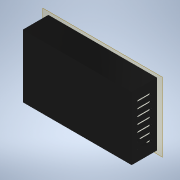
# Autodesk Inventor part: HANDHELD_BOTTOM
Saved by Autodesk Inventor 2020 (Build 240168000, 168)
## iProperties
Created: 2023-03-16
Part Number: HANDHELD_BOTTOM
Material: PC/ABS Plastic
Document SubType Name: Modeling
Designer: catsm
Density: 0.357273 g/cm^3
Appearance: Smooth - White
Author: catsm
Autodesk Inventor part; units mm, degrees
ref_plane "YZ Plane" through (0, 0, 0) normal (1, 0, 0) x (0, 1, 0)
ref_plane "XZ Plane" through (0, 0, 0) normal (0, 1, 0) x (-1, 0, 0)
ref_plane "Work Plane1" through (0, 0, 0) normal (0, 0, 1) x (1, 0, 0)
sketch "Sketch1" plane through (0, 0, 0) normal (0, 0, 1) x (1, 0, 0)
  line L0 (-101.8665, 59.0165) -> (-101.8665, -59.0165) projected
  line L1 (101.8665, 59.0165) -> (-101.8665, 59.0165) projected
  line L2 (101.8665, -59.0165) -> (101.8665, 59.0165) projected
  line L3 (-101.8665, -59.0165) -> (101.8665, -59.0165) projected
  line L4 (-98.6915, 55.8415) -> (-98.6915, -55.8415)
  line L5 (-98.6915, -55.8415) -> (98.6915, -55.8415)
  line L6 (98.6915, -55.8415) -> (98.6915, 55.8415)
  line L7 (98.6915, 55.8415) -> (-98.6915, 55.8415)
  point P0 (0, 0)
  dimension "d0" = 3.175
  constraints: 8 end point, 3 other
  measures "d0" distance between parallel lines of L1 L7
extrude "Extrusion1" add sketch "Sketch1" along normal blind 44.45
sketch "Sketch2" plane through (101.8665, -59.0165, 0) normal (1, 0, 0) x (0, 0, -1)
  circle A0 centre (-3.048, 109.9558) radius 1.905 projected
  circle A1 centre (-3.048, 8.0772) radius 1.778 projected
  circle A2 centre (-3.048, 8.0772) radius 1.016
  circle A3 centre (-3.048, 109.9558) radius 1.016
  point P0 (0, 59.0165)
  dimension "d3" = 2.032
  dimension "d4" = 2.032
  constraints: 2 centre point, 2 coincident
  measures "d3" diameter of A2
  measures "d4" diameter of A3
extrude "Extrusion2" cut sketch "Sketch2" against normal up to surface (203.733 mm away) contours A2 | A3
sketch "Sketch3" plane through (0, 0, 44.45) normal (0, 0, 1) x (1, 0, 0)
  line L0 (101.8665, 59.0165) -> (-101.8665, 59.0165) projected
  line L1 (-101.8665, 59.0165) -> (-101.8665, -59.0165) projected
  line L2 (-101.8665, -59.0165) -> (101.8665, -59.0165) projected
  line L3 (101.8665, -59.0165) -> (101.8665, 59.0165) projected
  line L4 (-98.6915, 55.8415) -> (98.6915, 55.8415) projected
  line L5 (98.6915, 55.8415) -> (98.6915, -55.8415) projected
  line L6 (98.6915, -55.8415) -> (-98.6915, -55.8415) projected
  line L7 (-98.6915, -55.8415) -> (-98.6915, 55.8415) projected
  point P0 (0, 0)
extrude "Extrusion3" add sketch "Sketch3" along normal blind 3.175 contours L3 L2 L1 L0 | L4 L5 L6 L7
sketch "Sketch4" plane through (0, 0, 44.45) normal (0, 0, -1) x (-1, 0, 0)
  circle A0 centre (93.7487, 50.8987) radius 1.5 projected
  circle A1 centre (93.7487, -40.5657) radius 1.5 projected
  circle A2 centre (38.7843, -40.5657) radius 1.5 projected
  circle A3 centre (38.7843, 50.8987) radius 1.5 projected
  circle A4 centre (93.7487, 50.8987) radius 3.556
  circle A5 centre (38.7843, 50.8987) radius 3.556
  circle A6 centre (38.7843, -40.5657) radius 3.556
  circle A7 centre (93.7487, -40.5657) radius 3.556
  point P0 (0, 0)
  dimension "d9" = 7.112
  dimension "d22" = 7.112
  dimension "d23" = 7.112
  dimension "d24" = 7.112
  constraints: 4 centre point, 1 coincident
  measures "d9" diameter of A4
  measures "d22" diameter of A5
  measures "d23" diameter of A6
  measures "d24" diameter of A7
ref_plane "Work Plane2" through (37.0165, -42.3335, 36.6431) normal (0, 0, 1) x (1, 0, 0)
extrude "Extrusion4" add sketch "Sketch4" along normal up to surface (7.8069 mm away) contours A0 | A1 | A2 | A3 | A4 | A5 | A6 | A7
sketch "Sketch6" plane through (-38.7843, -40.5657, 36.6431) normal (0, 0, -1) x (-1, 0, 0)
  circle A0 centre (0, 0) radius 1.5 projected
  circle A1 centre (54.9645, 0) radius 1.5 projected
  circle A2 centre (54.9645, 91.4645) radius 1.5 projected
  circle A3 centre (0, 91.4645) radius 1.5 projected
  circle A4 centre (54.9645, 91.4645) radius 3.556 projected
  point P0 (-38.7843, 40.5657)
  constraints: 4 coincident
hole "Hole2" at (-93.7487, 50.8987, 36.6431) at (-38.7843, 50.8987, 36.6431) at (-38.7843, -40.5657, 36.6431) at (-93.7487, -40.5657, 36.6431) direction (0, 0, 1) diameter 3.556 depth 7.8069 countersink diameter 3.81 countersink angle 82
sketch "Sketch7" plane through (0, 0, 44.45) normal (0, 0, -1) x (-1, 0, 0)
  line L0 (22.0258, -44.3326) -> (21.8153, -44.3326) projected
  line L1 (22.3278, -44.8451) -> (22.3278, -44.6284) projected
  line L2 (15.6236, -51.3326) -> (15.8403, -51.3326) projected
  line L3 (15.3278, -50.8201) -> (15.3278, -51.0306) projected
  line L4 (22.3278, -44.3326) -> (15.3278, -44.3326)
  line L5 (15.3278, -44.3326) -> (15.3278, -51.3326)
  line L6 (15.3278, -51.3326) -> (22.3278, -51.3326)
  line L7 (22.3278, -51.3326) -> (22.3278, -44.3326)
  line L8 (23.3044, -47.8326) -> (14.4144, -47.8326) construction
  line L9 (23.3044, -44.6576) -> (14.4144, -44.6576)
  line L10 (14.4144, -51.0076) -> (23.3044, -51.0076)
  arc A0 (23.3044, -51.0076) -> (23.3044, -44.6576) centre (23.3044, -47.8326) ccw
  arc A1 (14.4144, -44.6576) -> (14.4144, -51.0076) centre (14.4144, -47.8326) ccw
  line L11 (26.4794, -38.1722) -> (26.4794, -56.2222) projected
  line L12 (11.2394, -56.2222) -> (11.2394, -38.1722) projected
  point P0 (0, 0)
  point P1 (18.8594, -47.8326)
  dimension "d32" = 6.35
  dimension "d33" = 3.175
  dimension "d34" = 3.175
  constraints: 16 end point, 4 point on circle, 4 tangent, 3 parallel, 2 centre point, 2 perpendicular, 1 horizontal, 1 midpoint
  measures "d32" diameter of A1
  measures "d33" distance from line of L11 L8.start
  measures "d34" distance from line of L12 L8.end
extrude "Extrusion5" add sketch "Sketch7" along normal blind 6.35 contours L9 L1 L7 L10 L3 L5 | L5 L3 L10 A1 L9 | L9 A0 L10 L7 L1
sketch "Sketch8" plane through (-98.6915, -55.8415, 0) normal (0, 1, 0) x (1, 0, 0)
  line L0 (87.4521, -37.1) -> (87.4521, -35.5) projected
  line L1 (86.9521, -35.5) -> (72.7121, -35.5) projected
  line L2 (86.9521, -37.1) -> (72.7121, -37.1) projected
  line L3 (72.2121, -37.1) -> (72.2121, -35.5) projected
  line L4 (87.4521, -35.5) -> (87.4521, -37.1) projected
  line L5 (72.2121, -35.5) -> (87.4521, -35.5)
  line L6 (87.4521, -35.5) -> (87.4521, -37.1)
  line L7 (87.4521, -37.1) -> (72.2121, -37.1)
  line L8 (72.2121, -37.1) -> (72.2121, -35.5)
  line L9 (87.7061, -35.246) -> (71.9581, -35.246)
  line L10 (71.9581, -35.246) -> (71.9581, -37.354)
  line L11 (71.9581, -37.354) -> (87.7061, -37.354)
  line L12 (87.7061, -37.354) -> (87.7061, -35.246)
  point P0 (98.6915, 0)
  dimension "d37" = 0.254
  constraints: 16 end point, 4 parallel, 2 perpendicular, 1 horizontal, 3 other
  measures "d37" distance between parallel lines of L5 L9
extrude "Extrusion6" cut sketch "Sketch8" against normal blind 1.143 contours L7 L2 L3 L5 L1 L0 | L12 L11 L10 L9
sketch "Sketch9" plane through (-101.8665, -59.0165, 0) normal (0, -1, 0) x (1, 0, 0)
  line L0 (89.9919, 33.75) -> (89.9919, 35.4) projected
  line L1 (75.9919, 33.75) -> (75.9919, 35.4) projected
  line L2 (77.3919, 33.65) -> (76.0919, 33.65) projected
  line L3 (76.1819, 35.5) -> (77.3919, 35.5) projected
  line L4 (75.9919, 35.5) -> (89.9919, 35.5)
  line L5 (89.9919, 35.5) -> (89.9919, 33.65)
  line L6 (89.9919, 33.65) -> (75.9919, 33.65)
  line L7 (75.9919, 33.65) -> (75.9919, 35.5)
  line L8 (75.7379, 33.396) -> (90.2459, 33.396)
  line L9 (90.2459, 33.396) -> (90.2459, 35.754)
  line L10 (90.2459, 35.754) -> (75.7379, 35.754)
  line L11 (75.7379, 35.754) -> (75.7379, 33.396)
  point P0 (101.8665, 0)
  dimension "d40" = 0.254
  constraints: 16 end point, 4 parallel, 2 perpendicular, 2 point on line, 1 horizontal, 3 other
  measures "d40" distance between parallel lines of L6 L8
extrude "Extrusion7" cut sketch "Sketch9" against normal up to surface (3.175 mm away) contours L5 L6 L2 L7 L1 L4 L3 L0 | L11 L10 L9 L8
sketch "Sketch10" plane through (-101.8665, -59.0165, 0) normal (0, -1, 0) x (1, 0, 0)
  line L0 (90.2459, 35.754) -> (90.2459, 33.396) projected
  line L1 (90.2459, 33.396) -> (75.7379, 33.396) projected
  line L2 (75.7379, 33.396) -> (75.7379, 35.754) projected
  line L3 (75.7379, 35.754) -> (90.2459, 35.754) projected
  line L4 (0, 0) -> (203.733, 0) projected
  line L5 (203.733, 0) -> (203.733, 47.625) projected
  line L6 (0, 47.625) -> (203.733, 47.625) projected
  line L7 (0, 0) -> (0, 47.625) projected
  line L8 (72.5629, 30.221) -> (93.4209, 30.221)
  line L9 (93.4209, 30.221) -> (93.4209, 38.929)
  line L10 (93.4209, 38.929) -> (72.5629, 38.929)
  line L11 (72.5629, 38.929) -> (72.5629, 30.221)
  point P0 (101.8665, 0)
  dimension "d43" = 3.175
  constraints: 8 end point, 3 other
  measures "d43" distance between parallel lines of L1 L8
extrude "Extrusion8" cut sketch "Sketch10" against normal blind 1.5875 contours L11 L10 L9 L8
sketch "Sketch11" plane through (0, 0, 44.45) normal (0, 0, -1) x (-1, 0, 0)
  line L0 (-82.4355, -55.2065) -> (-82.4355, -39.2045) projected
  line L1 (-92.3415, -39.2045) -> (-92.3415, -55.2065) projected
  line L2 (-84.023, -48.412) -> (-90.754, -48.412) construction
  line L3 (-84.023, -46.8245) -> (-90.754, -46.8245)
  line L4 (-90.754, -49.9995) -> (-84.023, -49.9995)
  arc A0 (-84.023, -49.9995) -> (-84.023, -46.8245) centre (-84.023, -48.412) ccw
  arc A1 (-90.754, -46.8245) -> (-90.754, -49.9995) centre (-90.754, -48.412) ccw
  line L5 (-98.6915, 55.8415) -> (-98.6915, -55.8415) projected
  line L6 (-98.6915, -55.8415) -> (98.6915, -55.8415) projected
  point P0 (0, 0)
  point P1 (-87.3885, -48.412)
  dimension "d49" = 1.5875
  dimension "d50" = 1.5875
  dimension "d51" = 1.5875
  dimension "d52" = 7.62
  dimension "d92" = 7.9375
  dimension "d93" = 7.4295
  constraints: 8 end point, 4 point on circle, 4 tangent, 2 centre point, 1 horizontal, 1 midpoint, 1 parallel
  measures "d49" distance from line of L1 L2.end
  measures "d50" distance from line of L0 L2.start
  measures "d51" radius of A0
  measures "d52" distance from line of L1.start L3
  measures "d92" distance from line of L5 L2.end
  measures "d93" distance from line of L6 L2.end
extrude "Extrusion9" add sketch "Sketch11" along normal blind 6.35
sketch "Sketch17" plane through (-101.8665, -59.0165, 0) normal (0, -1, 0) x (1, 0, 0)
  line L0 (184.8894, 33.1978) -> (193.6206, 33.1978) projected
  line L1 (193.6206, 36.3728) -> (184.8894, 36.3728) projected
  line L2 (193.6206, 33.1978) -> (193.6206, 36.3728) projected
  line L3 (72.5629, 30.221) -> (72.5629, 38.929) projected
  line L4 (72.5629, 38.929) -> (93.4209, 38.929) projected
  line L5 (93.4209, 38.929) -> (93.4209, 30.221) projected
  line L6 (93.4209, 30.221) -> (72.5629, 30.221) projected
  line L7 (0, 0) -> (203.733, 0) projected
  line L8 (203.733, 0) -> (203.733, 47.625) projected
  line L9 (0, 47.625) -> (203.733, 47.625) projected
  line L10 (0, 0) -> (0, 47.625) projected
  line L11 (184.8894, 36.3728) -> (184.8894, 33.1978) projected
  line L12 (184.302, 38.1) -> (184.302, 36.5252) projected
  line L13 (194.208, 38.1) -> (194.208, 36.5252) projected
  line L14 (194.208, 38.1) -> (184.302, 38.1) projected
  line L15 (193.8746, 32.9438) -> (184.6354, 32.9438)
  line L16 (184.6354, 32.9438) -> (184.6354, 36.6268)
  line L17 (184.6354, 36.6268) -> (193.8746, 36.6268)
  line L18 (193.8746, 36.6268) -> (193.8746, 32.9438)
  point P0 (101.8665, 0)
  dimension "d74" = 0.254
  constraints: 8 end point, 3 other
  measures "d74" distance between parallel lines of L0 L15
extrude "Extrusion15" cut sketch "Sketch17" against normal up to surface (3.175 mm away) contours L11 L1 L2 L0 | L15 L16 L17 L18
sketch "Sketch18" plane through (-101.8665, -59.0165, 0) normal (0, -1, 0) x (1, 0, 0)
  line L0 (184.6354, 36.6268) -> (193.8746, 36.6268) projected
  line L1 (193.8746, 36.6268) -> (193.8746, 32.9438) projected
  line L2 (193.8746, 32.9438) -> (184.6354, 32.9438) projected
  line L3 (184.6354, 32.9438) -> (184.6354, 36.6268) projected
  line L4 (72.5629, 30.221) -> (72.5629, 38.929) projected
  line L5 (72.5629, 38.929) -> (93.4209, 38.929) projected
  line L6 (93.4209, 38.929) -> (93.4209, 30.221) projected
  line L7 (93.4209, 30.221) -> (72.5629, 30.221) projected
  line L8 (0, 0) -> (203.733, 0) projected
  line L9 (203.733, 0) -> (203.733, 47.625) projected
  line L10 (0, 47.625) -> (203.733, 47.625) projected
  line L11 (0, 0) -> (0, 47.625) projected
  line L12 (183.0479, 31.3563) -> (195.4621, 31.3563)
  line L13 (195.4621, 31.3563) -> (195.4621, 38.2143)
  line L14 (195.4621, 38.2143) -> (183.0479, 38.2143)
  line L15 (183.0479, 38.2143) -> (183.0479, 31.3563)
  point P0 (101.8665, 0)
  dimension "d77" = 1.5875
  constraints: 8 end point, 3 other
  measures "d77" distance between parallel lines of L2 L12
extrude "Extrusion16" cut sketch "Sketch18" against normal blind 1.5875 contours L15 L14 L13 L12
sketch "Sketch19" plane through (-101.8665, -59.0165, 0) normal (0, -1, 0) x (1, 0, 0)
  line L0 (183.0479, 31.3563) -> (183.0479, 38.2143) projected
  line L1 (184.6354, 36.6268) -> (184.6354, 32.9438) projected
  line L2 (184.6354, 36.6268) -> (184.6354, 32.9438) projected
  line L3 (184.6354, 34.7853) -> (183.0479, 34.7853)
  line L4 (183.0479, 31.3563) -> (183.0479, 38.2143) projected
  circle A0 centre (176.6979, 34.7853) radius 2.54
  circle A1 centre (167.1729, 34.7853) radius 2.54
  circle A2 centre (157.6479, 34.7853) radius 3.175
  point P0 (101.8665, 0)
  dimension "d80" = 5.08
  dimension "d81" = 5.08
  dimension "d82" = 6.35
  dimension "d83" = 0
  dimension "d84" = 6.35
  dimension "d85" = 9.525
  dimension "d86" = 9.525
  constraints: 3 centre point, 2 end point, 2 horizontal alignment, 2 midpoint
  measures "d80" diameter of A0
  measures "d81" diameter of A1
  measures "d82" diameter of A2
  measures "d83" distance from line of L3 A0.centre
  measures "d84" distance from line of L0 A0.centre
  measures "d85" distance of A1.centre A0.centre
  measures "d86" distance of A1.centre A2.centre
extrude "Extrusion17" cut sketch "Sketch19" against normal up to surface (3.175 mm away)
sketch "Sketch20" plane through (-101.8665, -59.0165, 0) normal (0, -1, 0) x (1, 0, 0)
  circle A0 centre (157.6479, 34.7853) radius 3.175 projected
  circle A1 centre (157.6479, 34.7853) radius 5.715
  point P0 (101.8665, 0)
  dimension "d89" = 2.54
  constraints: 1 centre point
  measures "d89" radial gap between concentric circles of A0 A1
extrude "Extrusion18" cut sketch "Sketch20" against normal blind 1.5875
sketch "Sketch21" plane through (101.8665, -59.0165, 0) normal (1, 0, 0) x (0, 0, -1)
  line L0 (-34.925, 59.0165) -> (-12.7, 59.0165) construction
  line L1 (-34.925, 56.4765) -> (-12.7, 56.4765)
  line L2 (-12.7, 61.5565) -> (-34.925, 61.5565)
  arc A0 (-34.925, 61.5565) -> (-34.925, 56.4765) centre (-34.925, 59.0165) ccw
  arc A1 (-12.7, 56.4765) -> (-12.7, 61.5565) centre (-12.7, 59.0165) ccw
  line L3 (0, 0) -> (0, 118.033) projected
  line L4 (-47.625, 0) -> (-47.625, 118.033) projected
  circle A2 centre (-3.048, 109.9558) radius 1.016 projected
  circle A3 centre (-3.048, 8.0772) radius 1.016 projected
  line L5 (0, 0) -> (0, 118.033) projected
  line L6 (0, 118.033) -> (-47.625, 118.033) projected
  line L7 (-47.625, 0) -> (-47.625, 118.033) projected
  line L8 (0, 0) -> (-47.625, 0) projected
  line L9 (-34.925, 69.1765) -> (-12.7, 69.1765)
  arc A4 (-12.7, 69.1765) -> (-12.7, 74.2565) centre (-12.7, 71.7165) ccw
  line L10 (-12.7, 74.2565) -> (-34.925, 74.2565)
  arc A5 (-34.925, 74.2565) -> (-34.925, 69.1765) centre (-34.925, 71.7165) ccw
  line L11 (-34.925, 81.8765) -> (-12.7, 81.8765)
  arc A6 (-12.7, 81.8765) -> (-12.7, 86.9565) centre (-12.7, 84.4165) ccw
  line L12 (-12.7, 86.9565) -> (-34.925, 86.9565)
  arc A7 (-34.925, 86.9565) -> (-34.925, 81.8765) centre (-34.925, 84.4165) ccw
  line L13 (-34.925, 94.5765) -> (-12.7, 94.5765)
  arc A8 (-12.7, 94.5765) -> (-12.7, 99.6565) centre (-12.7, 97.1165) ccw
  line L14 (-12.7, 99.6565) -> (-34.925, 99.6565)
  arc A9 (-34.925, 99.6565) -> (-34.925, 94.5765) centre (-34.925, 97.1165) ccw
  line L15 (-34.925, 43.7765) -> (-12.7, 43.7765)
  arc A10 (-12.7, 43.7765) -> (-12.7, 48.8565) centre (-12.7, 46.3165) ccw
  line L16 (-12.7, 48.8565) -> (-34.925, 48.8565)
  arc A11 (-34.925, 48.8565) -> (-34.925, 43.7765) centre (-34.925, 46.3165) ccw
  line L17 (-34.925, 56.4765) -> (-12.7, 56.4765)
  arc A12 (-12.7, 56.4765) -> (-12.7, 61.5565) centre (-12.7, 59.0165) ccw
  line L18 (-12.7, 61.5565) -> (-34.925, 61.5565)
  arc A13 (-34.925, 61.5565) -> (-34.925, 56.4765) centre (-34.925, 59.0165) ccw
  line L19 (-34.925, 69.1765) -> (-12.7, 69.1765)
  arc A14 (-12.7, 69.1765) -> (-12.7, 74.2565) centre (-12.7, 71.7165) ccw
  line L20 (-12.7, 74.2565) -> (-34.925, 74.2565)
  arc A15 (-34.925, 74.2565) -> (-34.925, 69.1765) centre (-34.925, 71.7165) ccw
  line L21 (-34.925, 81.8765) -> (-12.7, 81.8765)
  arc A16 (-12.7, 81.8765) -> (-12.7, 86.9565) centre (-12.7, 84.4165) ccw
  line L22 (-12.7, 86.9565) -> (-34.925, 86.9565)
  arc A17 (-34.925, 86.9565) -> (-34.925, 81.8765) centre (-34.925, 84.4165) ccw
  line L23 (-34.925, 31.0765) -> (-12.7, 31.0765)
  arc A18 (-12.7, 31.0765) -> (-12.7, 36.1565) centre (-12.7, 33.6165) ccw
  line L24 (-12.7, 36.1565) -> (-34.925, 36.1565)
  arc A19 (-34.925, 36.1565) -> (-34.925, 31.0765) centre (-34.925, 33.6165) ccw
  line L25 (-34.925, 43.7765) -> (-12.7, 43.7765)
  arc A20 (-12.7, 43.7765) -> (-12.7, 48.8565) centre (-12.7, 46.3165) ccw
  line L26 (-12.7, 48.8565) -> (-34.925, 48.8565)
  arc A21 (-34.925, 48.8565) -> (-34.925, 43.7765) centre (-34.925, 46.3165) ccw
  line L27 (-34.925, 56.4765) -> (-12.7, 56.4765)
  arc A22 (-12.7, 56.4765) -> (-12.7, 61.5565) centre (-12.7, 59.0165) ccw
  line L28 (-12.7, 61.5565) -> (-34.925, 61.5565)
  arc A23 (-34.925, 61.5565) -> (-34.925, 56.4765) centre (-34.925, 59.0165) ccw
  line L29 (-34.925, 69.1765) -> (-12.7, 69.1765)
  arc A24 (-12.7, 69.1765) -> (-12.7, 74.2565) centre (-12.7, 71.7165) ccw
  line L30 (-12.7, 74.2565) -> (-34.925, 74.2565)
  arc A25 (-34.925, 74.2565) -> (-34.925, 69.1765) centre (-34.925, 71.7165) ccw
  line L31 (-34.925, 18.3765) -> (-12.7, 18.3765)
  arc A26 (-12.7, 18.3765) -> (-12.7, 23.4565) centre (-12.7, 20.9165) ccw
  line L32 (-12.7, 23.4565) -> (-34.925, 23.4565)
  arc A27 (-34.925, 23.4565) -> (-34.925, 18.3765) centre (-34.925, 20.9165) ccw
  line L33 (-34.925, 31.0765) -> (-12.7, 31.0765)
  arc A28 (-12.7, 31.0765) -> (-12.7, 36.1565) centre (-12.7, 33.6165) ccw
  line L34 (-12.7, 36.1565) -> (-34.925, 36.1565)
  arc A29 (-34.925, 36.1565) -> (-34.925, 31.0765) centre (-34.925, 33.6165) ccw
  line L35 (-34.925, 43.7765) -> (-12.7, 43.7765)
  arc A30 (-12.7, 43.7765) -> (-12.7, 48.8565) centre (-12.7, 46.3165) ccw
  line L36 (-12.7, 48.8565) -> (-34.925, 48.8565)
  arc A31 (-34.925, 48.8565) -> (-34.925, 43.7765) centre (-34.925, 46.3165) ccw
  line L37 (-34.925, 56.4765) -> (-12.7, 56.4765)
  arc A32 (-12.7, 56.4765) -> (-12.7, 61.5565) centre (-12.7, 59.0165) ccw
  line L38 (-12.7, 61.5565) -> (-34.925, 61.5565)
  arc A33 (-34.925, 61.5565) -> (-34.925, 56.4765) centre (-34.925, 59.0165) ccw
  point P0 (0, 59.0165)
  point P1 (-23.8125, 59.0165)
  dimension "d95" = 5.08
  dimension "d96" = 12.7
  dimension "d97" = 12.7
  dimension "d98" = 0
  dimension "d101" = 12.7
  dimension "d104" = 12.7
  constraints: 68 end point, 64 point on circle, 32 centre point, 4 tangent, 2 vertical, 1 horizontal, 1 midpoint, 1 parallel, 150 other
  measures "d95" diameter of A1
  measures "d96" distance from line of L3 L0.end
  measures "d97" distance from line of L4 L0.start
  measures "d98" vertical distance of point (0, 59.017) point (-23.812, 59.017)
  measures "d101" distance of L1.start L9.start
  measures "d104" distance of L1.start L15.start
extrude "Extrusion19" cut sketch "Sketch21" against normal up to surface (3.175 mm away) contours A0 L2 A1 L1 | A5 L10 A4 L9 | A7 L12 A6 L11 | A9 L14 A8 L13 | A11 L16 A10 L15 | A19 L24 A18 L23 | A27 L32 A26 L31
sketch "Sketch22" plane through (-101.8665, -59.0165, 0) normal (-1, 0, 0) x (0, 0, 1)
  line L0 (34.925, 48.8565) -> (12.7, 48.8565) projected
  arc A0 (12.7, 48.8565) -> (12.7, 43.7765) centre (12.7, 46.3165) ccw projected
  line L1 (12.7, 43.7765) -> (34.925, 43.7765) projected
  arc A1 (34.925, 43.7765) -> (34.925, 48.8565) centre (34.925, 46.3165) ccw projected
  line L2 (34.925, 23.4565) -> (12.7, 23.4565) projected
  arc A2 (12.7, 23.4565) -> (12.7, 18.3765) centre (12.7, 20.9165) ccw projected
  line L3 (12.7, 18.3765) -> (34.925, 18.3765) projected
  arc A3 (34.925, 18.3765) -> (34.925, 23.4565) centre (34.925, 20.9165) ccw projected
  arc A4 (34.925, 69.1765) -> (34.925, 74.2565) centre (34.925, 71.7165) ccw projected
  line L4 (34.925, 74.2565) -> (12.7, 74.2565) projected
  arc A5 (12.7, 74.2565) -> (12.7, 69.1765) centre (12.7, 71.7165) ccw projected
  line L5 (12.7, 69.1765) -> (34.925, 69.1765) projected
  line L6 (12.7, 81.8765) -> (34.925, 81.8765) projected
  arc A6 (34.925, 81.8765) -> (34.925, 86.9565) centre (34.925, 84.4165) ccw projected
  line L7 (34.925, 86.9565) -> (12.7, 86.9565) projected
  arc A7 (12.7, 86.9565) -> (12.7, 81.8765) centre (12.7, 84.4165) ccw projected
  line L8 (34.925, 36.1565) -> (12.7, 36.1565) projected
  arc A8 (12.7, 36.1565) -> (12.7, 31.0765) centre (12.7, 33.6165) ccw projected
  line L9 (12.7, 31.0765) -> (34.925, 31.0765) projected
  arc A9 (34.925, 31.0765) -> (34.925, 36.1565) centre (34.925, 33.6165) ccw projected
  line L10 (12.7, 56.4765) -> (34.925, 56.4765) projected
  arc A10 (34.925, 56.4765) -> (34.925, 61.5565) centre (34.925, 59.0165) ccw projected
  line L11 (34.925, 61.5565) -> (12.7, 61.5565) projected
  arc A11 (12.7, 61.5565) -> (12.7, 56.4765) centre (12.7, 59.0165) ccw projected
  line L12 (12.7, 94.5765) -> (34.925, 94.5765) projected
  arc A12 (34.925, 94.5765) -> (34.925, 99.6565) centre (34.925, 97.1165) ccw projected
  line L13 (34.925, 99.6565) -> (12.7, 99.6565) projected
  arc A13 (12.7, 99.6565) -> (12.7, 94.5765) centre (12.7, 97.1165) ccw projected
  circle A14 centre (3.048, 109.9558) radius 1.016 projected
  circle A15 centre (3.048, 8.0772) radius 1.016 projected
  line L14 (0, 0) -> (0, 118.033) projected
  line L15 (0, 118.033) -> (47.625, 118.033) projected
  line L16 (47.625, 0) -> (47.625, 118.033) projected
  line L17 (0, 0) -> (47.625, 0) projected
  point P0 (0, 59.0165)
extrude "Extrusion20" cut sketch "Sketch22" against normal up to surface (3.175 mm away) contours A1 L1 A0 L0 | A3 L3 A2 L2 | L5 A5 L4 A4 | A7 L7 A6 L6 | A9 L9 A8 L8 | A11 L11 A10 L10 | A13 L13 A12 L12
body "Solid1"
